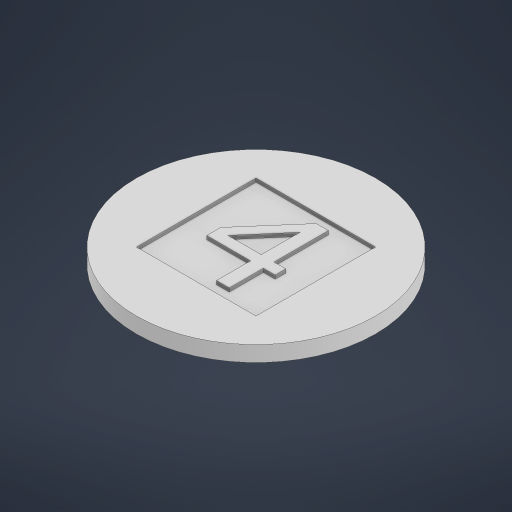
# Autodesk Inventor part: TopMarker4
Saved by Autodesk Inventor 2023 (Build 270158000, 158)
## iProperties
Created: 2023-03-04
Part Number: TopMarker4
Material: Generic
Document SubType Name: Modeling
Designer: Elias Braun
Density: 1 g/cm^3
Appearance: Default
Author: Elias Braun
Autodesk Inventor part; units mm, degrees
ref_plane "YZ Plane" through (0, 0, 0) normal (1, 0, 0) x (0, 1, 0)
ref_plane "XZ Plane" through (0, 0, 0) normal (0, 1, 0) x (-1, 0, 0)
ref_plane "XY Plane" through (0, 0, 0) normal (0, 0, 1) x (1, 0, 0)
sketch "Sketch1" plane through (0, 0, 0) normal (0, 1, 0) x (-1, 0, 0)
  circle A0 centre (0, 0) radius 20
  dimension "d0" = 40
  constraints: 1 centre point, 1 coincident
  measures "d0" diameter of A0
extrude "Extrusion1" add sketch "Sketch1" along normal blind 2.6
sketch "Sketch2" plane through (0, 2.6, 0) normal (0, 1, 0) x (1, 0, 0)
  line L0 (-10, -10) -> (-10, 10)
  line L1 (-10, 10) -> (10, 10)
  line L2 (10, 10) -> (10, -10)
  line L3 (10, -10) -> (-10, -10)
  line L4 (-10, -10) -> (10, 10) construction
  line L5 (-10, 10) -> (10, -10) construction
  point P0 (0, 0)
  dimension "d3" = 20
  dimension "d4" = 20
  constraints: 12 end point, 2 midpoint, 2 parallel, 1 perpendicular, 1 vertical
  measures "d3" distance of L0.start L0.end
  measures "d4" distance of L0.end L1.end
extrude "Extrusion2" cut sketch "Sketch2" against normal blind 0.6
sketch "Sketch3" plane through (0, 2, 0) normal (0, 1, 0) x (1, 0, 0)
  line L0 (-6.2284, 8.4382) -> (6.2284, 8.4382) construction
  line L1 (6.2284, 8.4382) -> (6.2284, -8.1618) construction
  line L2 (6.2284, -8.1618) -> (-6.2284, -8.1618) construction
  line L3 (-6.2284, -8.1618) -> (-6.2284, 8.4382) construction
  line L4 (5.6634, -2.4581) -> (3.6859, -2.4581)
  line L5 (3.6859, -2.4581) -> (3.6859, -8.1618)
  line L6 (3.6859, -8.1618) -> (1.547, -8.1618)
  line L7 (1.547, -8.1618) -> (1.547, -2.4581)
  line L8 (1.547, -2.4581) -> (-5.7844, -2.4581)
  line L9 (-5.7844, -2.4581) -> (-5.7844, -0.1174)
  line L10 (-5.7844, -0.1174) -> (1.6412, 8.4382)
  line L11 (1.6412, 8.4382) -> (3.6859, 8.4382)
  line L12 (3.6859, 8.4382) -> (3.6859, -0.6689)
  line L13 (3.6859, -0.6689) -> (5.6634, -0.6689)
  line L14 (5.6634, -0.6689) -> (5.6634, -2.4581)
  line L15 (1.547, -0.6689) -> (1.547, 5.815)
  line L16 (1.547, 5.815) -> (-4.0357, -0.6689)
  line L17 (-4.0357, -0.6689) -> (1.547, -0.6689)
  point P0 (0, 0)
  constraints: 2 other
extrude "Extrusion3" add sketch "Sketch3" along normal blind 0.6
body "Solid1"
